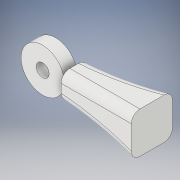
# Autodesk Inventor part: Arm4
Saved by Autodesk Inventor 2017 SP1 (Build 210196100, 196)
## iProperties
Created: 2018-02-11
Part Number: Arm4
Material: ABS Plastic
Document SubType Name: Modeling
Designer: Zach
Density: 1.06 g/cm^3
Appearance: CR White
Author: Zach
Autodesk Inventor part; units mm, degrees
ref_plane "YZ Plane" through (0, 0, 0) normal (1, 0, 0) x (0, 1, 0)
ref_plane "XZ Plane" through (0, 0, 0) normal (0, 1, 0) x (-1, 0, 0)
ref_plane "XY Plane" through (0, 0, 0) normal (0, 0, 1) x (1, 0, 0)
sketch "Sketch1" plane through (0, 0, 0) normal (0, 0, 1) x (1, 0, 0)
  circle A0 centre (0, 0) radius 1.5
  circle A1 centre (0, 0) radius 5
  dimension "d0" = 3
  dimension "d1" = 10
  constraints: 2 centre point, 2 coincident
  measures "d0" diameter of A0
  measures "d1" diameter of A1
extrude "Extrusion1" add sketch "Sketch1" along normal blind 3
sketch "Sketch2" plane through (0, 0, 3) normal (0, 0, 1) x (1, 0, 0)
  circle A0 centre (0, 0) radius 5 projected
  line L0 (4.7697, 1.5) -> (5.7697, 1.5)
  line L1 (5.7697, 1.5) -> (5.7697, -1.5)
  line L2 (5.7697, -1.5) -> (4.7697, -1.5)
  line L3 (4.7697, -1.5) -> (4.7697, 1.5)
  circle A1 centre (0, 0) radius 5 projected
  point P0 (4.7697, 0)
  dimension "d4" = 1
  dimension "d8" = 3
  constraints: 8 end point, 2 parallel, 1 horizontal, 1 horizontal alignment, 1 midpoint, 1 perpendicular, 4 other
  measures "d4" distance between parallel lines of L1 L3
  measures "d8" distance of L0.end L1.end
extrude "Extrusion2" add sketch "Sketch2" against normal blind 3 contours A0 L3 | A0 L0 L1 L2 picked at (4.8122, -0.3362)
sketch "Sketch3" plane through (5.7697, -1.5, 3) normal (1, 0, 0) x (0, 0, -1)
  line L0 (-1.5, 4.5) -> (4.5, 4.5)
  line L1 (4.5, 4.5) -> (4.5, -1.5)
  line L2 (4.5, -1.5) -> (-1.5, -1.5)
  line L3 (-1.5, -1.5) -> (-1.5, 4.5)
  line L4 (0, 3) -> (3, 3) projected
  line L5 (0, 3) -> (0, 0) projected
  point P0 (3, 1.5)
  point P1 (0, 1.5)
  point P2 (-1.5, 1.5)
  point P3 (1.5, 3)
  point P4 (1.5, 4.5)
  dimension "d9" = 6
  dimension "d10" = 6
  constraints: 8 end point, 4 midpoint, 2 parallel, 1 horizontal, 1 horizontal alignment, 1 perpendicular, 1 vertical alignment
  measures "d9" distance of L1.end L2.end
  measures "d10" distance of L0.end L1.end
extrude "Extrusion3" add sketch "Sketch3" along normal blind 18
sketch "Sketch4" plane through (5.7697, -3, 4.5) normal (0, 0, 1) x (1, 0, 0)
  line L0 (18, 7.75) -> (18, -1.75)
  line L1 (18, 6) -> (18, 0) projected
  line L2 (0, 0) -> (0, 6) projected
  arc A0 (0, 6) -> (18, 7.75) centre (-5.4885, 155.8996) ccw
  arc A1 (18, -1.75) -> (0, 0) centre (-5.4885, -149.8996) ccw
  line L3 (0, 0) -> (18, 0) projected
  line L4 (0, 0) -> (18, 0)
  line L5 (18, 0) -> (18, -1.75)
  line L6 (0, 6) -> (18, 6) projected
  line L7 (0, 6) -> (18, 6)
  line L8 (18, 6) -> (18, 7.75)
  point P0 (-5.7697, 3)
  point P1 (18, 3)
  dimension "d13" = 9.5
  dimension "d14" = 150
  dimension "d15" = 150
  constraints: 10 end point, 4 point on circle, 2 centre point, 2 collinear, 2 midpoint, 1 horizontal, 1 perpendicular, 1 vertical
  measures "d13" distance of L0.start L0.end
  measures "d14" radius of A0
  measures "d15" radius of A1
extrude "Extrusion4" add sketch "Sketch4" against normal blind 6 contours L0 L6 A0 | L0 A1 L3
sketch "Sketch5" plane through (4.7697, 1.5, 3) normal (0, 1, 0) x (1, 0, 0)
  line L0 (19, 6.25) -> (19, -3.25)
  line L1 (19, -1.5) -> (19, 4.5) projected
  arc A0 (1, 4.5) -> (19, 6.25) centre (-4.4885, 154.3996) ccw
  line L2 (19, -1.5) -> (1, -1.5) projected
  arc A1 (19, -3.25) -> (1, -1.5) centre (-4.4885, -151.3996) ccw
  line L3 (1, 4.5) -> (19, 4.5)
  line L4 (19, 4.5) -> (19, 6.25)
  line L5 (1, -1.5) -> (19, -1.5)
  line L6 (19, -1.5) -> (19, -3.25)
  point P0 (-4.7697, 3)
  point P1 (19, 1.5)
  dimension "d18" = 9.5
  dimension "d19" = 150
  dimension "d20" = 150
  constraints: 10 end point, 4 point on circle, 2 centre point, 2 collinear, 2 midpoint, 1 horizontal, 1 perpendicular, 1 vertical
  measures "d18" distance of L0.start L0.end
  measures "d19" radius of A0
  measures "d20" radius of A1
extrude "Extrusion5" add sketch "Sketch5" along normal blind 3.25 and the other way blind 6.25
sketch "Sketch6" plane through (5.7697, -4.75, -1.5) normal (0, 0, 1) x (1, 0, 0)
  arc A0 (0, 7.75) -> (18, 9.5) centre (-5.4885, 157.6496) ccw projected
  line L0 (0, 9.5) -> (18, 9.5) projected
  line L1 (0, 7.75) -> (0, 9.5) projected
  arc A1 (18, 0) -> (0, 1.75) centre (-5.4885, -148.1496) ccw projected
  line L2 (0, 0) -> (0, 1.75) projected
  line L3 (18, 0) -> (0, 0) projected
  point P0 (-5.7697, 4.75)
extrude "Extrusion6" cut sketch "Sketch6" along normal through all both and the other way through all
fillet "Fillet1" radius 2 4 edges at (14.7961, 3.6035, -2.1035) (14.872, 3.6109, 5.1109) (14.872, -3.6109, 5.1109) (14.7961, -3.6035, -2.1035)
body "Solid1"
